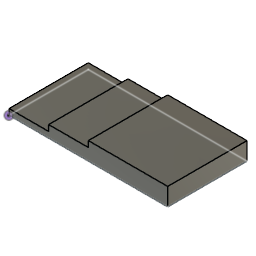
StaircaseF3D (Autodesk Fusion 360 design; units mm, degrees)
part number: 2026-06-30-23-35-38-396
Autodesk Fusion 360 part; units mm, degrees
sketch "Sketch1" plane through (0, 0, 0) normal (0, 0, 1) x (1, 0, 0)
  line L0 (0, 0) -> (800, 0)
  line L1 (800, 0) -> (800, 400)
  line L2 (800, 400) -> (0, 400)
  line L3 (0, 400) -> (0, 0)
  dimension "d1" = 800
  dimension "d2" = 400
  constraint horizontal L0
  constraint vertical L1
  constraint horizontal L2
  constraint vertical L3
  constraint coincident L0.start L3.end
  measures "d1" distance of L0.start L0.end
  measures "d2" distance of L0.start L2.end
extrude "Extrude1" add sketch "Sketch1" along normal blind 90
sketch "Sketch2" plane through (0, 0, 0) normal (-1, 0, 0) x (0, -1, 0)
  line L0 (-400, 0) -> (0, 0)
  line L1 (0, 0) -> (0, 90)
  line L2 (0, 90) -> (-400, 90)
  line L3 (-400, 90) -> (-400, 0)
  line L4 (-200, 90) -> (-200, 60) construction
  line L5 (-200, 60) -> (-200, 30) construction
  line L6 (-200, 30) -> (-200, 0) construction
  line L7 (-400, 90) -> (0, 90) construction
  line L8 (0, 90) -> (0, 60) construction
  line L9 (0, 60) -> (-400, 60)
  line L10 (-400, 60) -> (-400, 90) construction
  line L11 (-400, 60) -> (0, 60) construction
  line L12 (0, 60) -> (0, 30) construction
  line L13 (0, 30) -> (-400, 30)
  line L14 (-400, 30) -> (-400, 60) construction
  dimension "d5" = 30
  dimension "d6" = 30
  constraint midpoint L2 L4.start
  constraint perpendicular L0 L4
  constraint perpendicular L2 L5
  constraint perpendicular L0 L6
  constraint horizontal L7
  constraint vertical L8
  constraint horizontal L9
  constraint vertical L10
  constraint coincident L1 L8.end
  constraint coincident L2.end L3.start
  constraint horizontal L11
  constraint vertical L12
  constraint horizontal L13
  constraint vertical L14
  constraint coincident L1 L12.end
  measures "d5" distance of L4.start L4.end
  measures "d6" distance of L4.end L5.end
extrude "Extrude2" cut sketch "Sketch2" against normal blind 400 contours L1 L2 L3 L9
extrude "Extrude3" cut sketch "Sketch2" against normal blind 200 contours L1 L3 L9 L13
